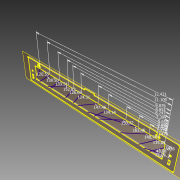
# Autodesk Inventor part: Panel_front
Saved by Autodesk Inventor 2013 (Build 170138000, 138)
## iProperties
Created: 2013-02-02
Part Number: Panel_front
Material: Aluminum 6061
Document SubType Name: Modeling
Designer: xylzlyx
Density: 1 g/cm^3
Author: xylzlyx
Autodesk Inventor part; units mm, degrees
ref_plane "YZ Plane" through (0, 0, 0) normal (1, 0, 0) x (0, 1, 0)
ref_plane "XZ Plane" through (0, 0, 0) normal (0, 1, 0) x (-1, 0, 0)
ref_plane "XY Plane" through (0, 0, 0) normal (0, 0, 1) x (1, 0, 0)
ref_plane "Work Plane1" through (0, 0, -9.525) normal (0, 0, 1) x (1, 0, 0)
sketch "Sketch1" plane through (0, 0, -9.525) normal (0, 0, 1) x (1, 0, 0)
  line L0 (381, -60.8043) -> (381, -64.0283) construction
  line L1 (381, -64.0283) -> (0, -64.0283) construction
  line L2 (0, -64.0283) -> (0, -60.8043) construction
  line L3 (0, -60.8043) -> (381, -60.8043) construction
  line L4 (381, 0) -> (0, 0) construction
  line L5 (0, 0) -> (0, 3.175) construction
  line L6 (0, 3.175) -> (381, 3.175) construction
  line L7 (381, 3.175) -> (381, 0) construction
  line L8 (381, -60.8043) -> (0, -60.8043)
  line L9 (0, -60.8043) -> (0, 0)
  line L10 (0, 0) -> (381, 0)
  line L11 (381, 0) -> (381, -60.8043)
  constraints: 24 end point, 5 horizontal, 4 coincident, 4 vertical, 2 parallel, 1 perpendicular, 8 other
extrude "FrontPanel" add sketch "Sketch1" against normal blind 3.175
fillet "CornerFillet" radius 1 4 edges at (381, -60.8043, -11.1125) (0, -60.8043, -11.1125) (0, 0, -11.1125) (381, 0, -11.1125)
sketch "ScrewSlotSketch" plane through (0, 0, -9.525) normal (0, 0, 1) x (1, 0, 0)
  line L0 (368.3, -28.0035) -> (368.3, -1) projected
  line L1 (12.7, -1) -> (12.7, -28.0035) projected
  line L2 (381, 0) -> (0, 0) construction
  line L3 (0, 0) -> (0, 3.175) construction
  line L4 (0, 3.175) -> (381, 3.175) construction
  line L5 (381, 3.175) -> (381, 0) construction
  line L6 (381, -60.8043) -> (381, -64.0283) construction
  line L7 (381, -64.0283) -> (0, -64.0283) construction
  line L8 (0, -64.0283) -> (0, -60.8043) construction
  line L9 (0, -60.8043) -> (381, -60.8043) construction
  line L10 (344.7987, -8.89) -> (344.7987, 3.175)
  line L11 (344.7987, 3.175) -> (341.0014, 3.175)
  line L12 (341.0014, 3.175) -> (341.0014, -8.89)
  line L13 (341.0014, -8.89) -> (344.7987, -8.89)
  line L14 (346.9958, -8.89) -> (338.8043, -8.89)
  line L15 (338.8043, -8.89) -> (338.8043, -5.8579)
  line L16 (338.8043, -5.8579) -> (346.9958, -5.8579)
  line L17 (346.9958, -5.8579) -> (346.9958, -8.89)
  line L18 (36.2014, -8.89) -> (39.9987, -8.89)
  line L19 (39.9987, -8.89) -> (39.9987, 3.175)
  line L20 (39.9987, 3.175) -> (36.2014, 3.175)
  line L21 (36.2014, 3.175) -> (36.2014, -8.89)
  line L22 (34.0043, -8.89) -> (42.1958, -8.89)
  line L23 (42.1958, -8.89) -> (42.1958, -5.8579)
  line L24 (42.1958, -5.8579) -> (34.0043, -5.8579)
  line L25 (34.0043, -5.8579) -> (34.0043, -8.89)
  point P0 (342.9, 3.175)
  point P1 (342.9, -8.89)
  point P2 (38.1, -8.89)
  point P3 (38.1, 3.175)
  dimension "d4" = 12.065
  dimension "d6" = 3.7973
  dimension "d7" = 25.4
  dimension "d8" = 8.1915
  dimension "d9" = 3.0321
  dimension "d10" = 3.7973
  dimension "d11" = 12.065
  dimension "d12" = 8.1915
  dimension "d13" = 3.0321
  dimension "d14" = 25.4
  constraints: 48 end point, 11 parallel, 6 horizontal, 6 midpoint, 4 vertical, 2 perpendicular, 2 point on line, 1 collinear, 7 other
  measures "d4" distance of L10.start L10.end
  measures "d6" distance of L10.end L11.end
  measures "d7" distance from line of L0 point (342.9, 3.175)
  measures "d8" distance of L14.start L14.end
  measures "d9" distance of L14.end L15.end
  measures "d10" distance of L19.end L20.end
  measures "d11" distance of L20.end L18.start
  measures "d12" distance of L22.start L22.end
  measures "d13" distance of L22.end L23.end
  measures "d14" distance from line of L1 point (38.1, 3.175)
extrude "ScrewSlotExtrusion" cut sketch "ScrewSlotSketch" against normal blind 3.175
fillet "ScrewSlotFillet" radius 0.5 16 edges at (344.7987, 0, -11.1125) (341.0014, 0, -11.1125) (344.7987, -5.8579, -11.1125) (341.0014, -5.8579, -11.1125) (338.8043, -5.8579, -11.1125) (338.8043, -8.89, -11.1125) (346.9958, -8.89, -11.1125) (346.9958, -5.8579, -11.1125) (42.1958, -8.89, -11.1125) (42.1958, -5.8579, -11.1125) (39.9987, -5.8579, -11.1125) (39.9987, 0, -11.1125) (36.2014, 0, -11.1125) (36.2014, -5.8579, -11.1125) (34.0043, -5.8579, -11.1125) (34.0043, -8.89, -11.1125)
sketch "ScrewHoleSketch" plane through (0, 0, -9.525) normal (0, 0, 1) x (1, 0, 0)
  line L0 (34.0043, -8.39) -> (34.0043, -6.3579) projected
  line L1 (368.3, -28.5035) -> (371.475, -28.5035) projected
  line L2 (371.475, -32.3008) -> (368.3, -32.3008) projected
  line L3 (9.525, -28.5035) -> (12.7, -28.5035) projected
  line L4 (12.7, -32.3008) -> (9.525, -32.3008) projected
  line L5 (371.475, -28.5035) -> (371.475, -32.3008) construction
  line L6 (9.525, -28.5035) -> (9.525, -32.3008) construction
  point P0 (0, 0)
  point P1 (11.1125, -30.4021)
  point P2 (369.8875, -30.4021)
  point P3 (369.8875, -28.5035)
  point P4 (371.475, -30.4021)
  point P5 (9.525, -30.4021)
  point P6 (11.1125, -28.5035)
  constraints: 4 end point, 4 midpoint, 2 horizontal alignment, 2 parallel, 2 vertical alignment
hole "ScrewHoles" at (11.1125, -30.4021, -9.525) at (369.8875, -30.4021, -9.525) direction (0, 0, -1) diameter 3.7973 end through all
sketch "BottomTabSketch" plane through (40.4987, 0, -9.525) normal (0, 1, 0) x (1, 0, 0)
  line L0 (162.7014, 3.175) -> (137.3014, 3.175)
  line L1 (137.3014, 3.175) -> (137.3014, 0)
  line L2 (137.3014, 0) -> (162.7014, 0)
  line L3 (162.7014, 0) -> (162.7014, 3.175)
  line L4 (137.0473, 2.929) -> (137.0473, 0.246) projected
  line L5 (137.5473, -0.254) -> (162.4553, -0.254) projected
  point P0 (0, 3.175)
  point P1 (-40.4987, -9.525)
  point P2 (137.3014, 1.5875)
  point P3 (137.0473, 1.5875)
  point P4 (150.0014, 0)
  point P5 (150.0013, -0.254)
  dimension "d29" = 25.4
  constraints: 8 end point, 4 midpoint, 2 horizontal alignment, 2 parallel, 1 horizontal, 1 perpendicular, 1 vertical alignment
  measures "d29" distance of L0.start L0.end
extrude "BottomTab" add sketch "BottomTabSketch" along normal blind 3.175
fillet "BottomTabFillet" radius 0.5 4 edges at (177.8, 0, -11.1125) (177.8, 3.175, -11.1125) (203.2, 3.175, -11.1125) (203.2, 0, -11.1125)
sketch "SlotSketch" plane through (0, 0, -9.525) normal (0, 0, 1) x (1, 0, 0)
  circle A0 centre (11.1125, -30.4021) radius 1.8986 projected
  circle A1 centre (369.8875, -30.4021) radius 1.8986 projected
  line L0 (371.729, -50.6197) -> (368.046, -50.6197)
  line L1 (368.046, -50.6197) -> (368.046, -40.5867)
  line L2 (368.046, -40.5867) -> (371.729, -40.5867)
  line L3 (371.729, -40.5867) -> (371.729, -50.6197)
  line L4 (12.954, -50.6197) -> (9.271, -50.6197)
  line L5 (9.271, -50.6197) -> (9.271, -40.5867)
  line L6 (9.271, -40.5867) -> (12.954, -40.5867)
  line L7 (12.954, -40.5867) -> (12.954, -50.6197)
  line L8 (380, -60.8043) -> (1, -60.8043) projected
  line L9 (203.2, 0.5) -> (203.2, 2.675) projected
  line L10 (11.1125, -30.4021) -> (11.1125, -60.8043) construction
  line L11 (369.8875, -30.4021) -> (369.8875, -60.8043) construction
  point P0 (0, 0)
  point P1 (12.954, -45.6032)
  point P2 (11.1125, -45.6032)
  point P3 (11.1125, -50.6197)
  point P4 (369.8875, -45.6032)
  point P5 (371.729, -45.6032)
  point P6 (369.8875, -50.6197)
  dimension "d34" = 10.033
  dimension "d36" = 3.683
  dimension "d37" = 10.033
  dimension "d38" = 3.683
  constraints: 20 end point, 6 midpoint, 6 parallel, 2 horizontal, 2 horizontal alignment, 2 perpendicular, 2 point on line, 2 vertical alignment
  measures "d34" distance of L0.end L1.end
  measures "d36" distance of L0.start L0.end
  measures "d37" distance of L6.end L4.start
  measures "d38" distance of L4.start L4.end
extrude "Extrusion4" cut sketch "SlotSketch" against normal blind 3.175 contours L0 L1 L2 L3 | L4 L5 L6 L7
fillet "Fillet5" radius 0.5 8 edges at (368.046, -40.5867, -11.1125) (371.729, -40.5867, -11.1125) (371.729, -50.6197, -11.1125) (368.046, -50.6197, -11.1125) (9.271, -40.5867, -11.1125) (12.954, -40.5867, -11.1125) (12.954, -50.6197, -11.1125) (9.271, -50.6197, -11.1125)
sketch "Sketch6" plane through (0, 0, -9.525) normal (0, 0, 1) x (1, 0, 0)
  line L0 (380, -60.8043) -> (1, -60.8043) projected
  line L1 (203.7, 0) -> (340.5014, 0) projected
  circle A0 centre (11.1125, -30.4021) radius 1.8986 projected
  circle A1 centre (369.8875, -30.4021) radius 1.8986 projected
  line L2 (357.1875, -48.1043) -> (23.8125, -48.1043)
  line L3 (23.8125, -48.1043) -> (23.8125, -12.7)
  line L4 (23.8125, -12.7) -> (357.1875, -12.7)
  line L5 (357.1875, -12.7) -> (357.1875, -48.1043)
  point P0 (0, 0)
  dimension "d42" = 12.7
  dimension "d43" = 12.7
  dimension "d44" = 12.7
  dimension "d45" = 12.7
  constraints: 8 end point, 2 parallel, 1 horizontal, 1 perpendicular
  measures "d42" distance from line of L0 L2.start
  measures "d43" distance between parallel lines of L1 L4
  measures "d44" distance from line of A1.centre L5
  measures "d45" distance from line of A0.centre L3
extrude "Extrusion5" cut sketch "Sketch6" against normal blind 25.4 contours L2 L3 L4 L5
fillet "Fillet6" radius 0.5 4 edges at (357.1875, -48.1043, -11.1125) (357.1875, -12.7, -11.1125) (23.8125, -48.1043, -11.1125) (23.8125, -12.7, -11.1125)
sketch "Sketch7" plane through (0, 0, -9.525) normal (0, 0, 1) x (1, 0, 0)
  line L0 (357.1875, -13.2) -> (357.1875, -47.6043) projected
  arc A0 (356.6875, -48.1043) -> (357.1875, -47.6043) centre (356.6875, -47.6043) ccw projected
  line L1 (356.6875, -48.1043) -> (24.3125, -48.1043) projected
  arc A1 (23.8125, -47.6043) -> (24.3125, -48.1043) centre (24.3125, -47.6043) ccw projected
  line L2 (23.8125, -47.6043) -> (23.8125, -13.2) projected
  arc A2 (24.3125, -12.7) -> (23.8125, -13.2) centre (24.3125, -13.2) ccw projected
  line L3 (24.3125, -12.7) -> (356.6875, -12.7) projected
  arc A3 (357.1875, -13.2) -> (356.6875, -12.7) centre (356.6875, -13.2) ccw projected
  line L4 (371.729, -41.0867) -> (371.729, -50.1197) projected
  arc A4 (371.229, -50.6197) -> (371.729, -50.1197) centre (371.229, -50.1197) ccw projected
  line L5 (371.229, -50.6197) -> (368.546, -50.6197) projected
  arc A5 (368.046, -50.1197) -> (368.546, -50.6197) centre (368.546, -50.1197) ccw projected
  line L6 (368.046, -50.1197) -> (368.046, -41.0867) projected
  arc A6 (368.546, -40.5867) -> (368.046, -41.0867) centre (368.546, -41.0867) ccw projected
  line L7 (368.546, -40.5867) -> (371.229, -40.5867) projected
  arc A7 (371.729, -41.0867) -> (371.229, -40.5867) centre (371.229, -41.0867) ccw projected
  line L8 (12.954, -41.0867) -> (12.954, -50.1197) projected
  arc A8 (12.454, -50.6197) -> (12.954, -50.1197) centre (12.454, -50.1197) ccw projected
  line L9 (12.454, -50.6197) -> (9.771, -50.6197) projected
  arc A9 (9.271, -50.1197) -> (9.771, -50.6197) centre (9.771, -50.1197) ccw projected
  line L10 (9.271, -50.1197) -> (9.271, -41.0867) projected
  arc A10 (9.771, -40.5867) -> (9.271, -41.0867) centre (9.771, -41.0867) ccw projected
  line L11 (9.771, -40.5867) -> (12.454, -40.5867) projected
  arc A11 (12.954, -41.0867) -> (12.454, -40.5867) centre (12.454, -41.0867) ccw projected
  arc A12 (203.2, 2.675) -> (202.7, 3.175) centre (202.7, 2.675) ccw projected
  line L12 (178.3, 3.175) -> (202.7, 3.175) projected
  arc A13 (178.3, 3.175) -> (177.8, 2.675) centre (178.3, 2.675) ccw projected
  line L13 (177.8, 0.5) -> (177.8, 2.675) projected
  arc A14 (177.3, 0) -> (177.8, 0.5) centre (177.3, 0.5) ccw projected
  line L14 (40.4987, 0) -> (177.3, 0) projected
  arc A15 (40.4987, 0) -> (39.9987, -0.5) centre (40.4987, -0.5) ccw projected
  line L15 (39.9987, -0.5) -> (39.9987, -5.3579) projected
  arc A16 (39.9987, -5.3579) -> (40.4987, -5.8579) centre (40.4987, -5.3579) ccw projected
  line L16 (40.4987, -5.8579) -> (41.6958, -5.8579) projected
  arc A17 (42.1958, -6.3579) -> (41.6958, -5.8579) centre (41.6958, -6.3579) ccw projected
  line L17 (42.1958, -6.3579) -> (42.1958, -8.39) projected
  arc A18 (41.6958, -8.89) -> (42.1958, -8.39) centre (41.6958, -8.39) ccw projected
  line L18 (41.6958, -8.89) -> (34.5043, -8.89) projected
  arc A19 (34.0043, -8.39) -> (34.5043, -8.89) centre (34.5043, -8.39) ccw projected
  line L19 (34.0043, -8.39) -> (34.0043, -6.3579) projected
  arc A20 (34.5043, -5.8579) -> (34.0043, -6.3579) centre (34.5043, -6.3579) ccw projected
  line L20 (34.5043, -5.8579) -> (35.7014, -5.8579) projected
  arc A21 (35.7014, -5.8579) -> (36.2014, -5.3579) centre (35.7014, -5.3579) ccw projected
  line L21 (36.2014, -5.3579) -> (36.2014, -0.5) projected
  arc A22 (36.2014, -0.5) -> (35.7014, 0) centre (35.7014, -0.5) ccw projected
  line L22 (1, 0) -> (35.7014, 0) projected
  arc A23 (1, 0) -> (0, -1) centre (1, -1) ccw projected
  line L23 (0, -59.8043) -> (0, -1) projected
  arc A24 (0, -59.8043) -> (1, -60.8043) centre (1, -59.8043) ccw projected
  line L24 (380, -60.8043) -> (1, -60.8043) projected
  arc A25 (380, -60.8043) -> (381, -59.8043) centre (380, -59.8043) ccw projected
  line L25 (381, -1) -> (381, -59.8043) projected
  arc A26 (381, -1) -> (380, 0) centre (380, -1) ccw projected
  line L26 (345.2987, 0) -> (380, 0) projected
  arc A27 (345.2987, 0) -> (344.7987, -0.5) centre (345.2987, -0.5) ccw projected
  line L27 (344.7987, -0.5) -> (344.7987, -5.3579) projected
  arc A28 (344.7987, -5.3579) -> (345.2987, -5.8579) centre (345.2987, -5.3579) ccw projected
  line L28 (345.2987, -5.8579) -> (346.4958, -5.8579) projected
  arc A29 (346.9958, -6.3579) -> (346.4958, -5.8579) centre (346.4958, -6.3579) ccw projected
  line L29 (346.9958, -6.3579) -> (346.9958, -8.39) projected
  arc A30 (346.4958, -8.89) -> (346.9958, -8.39) centre (346.4958, -8.39) ccw projected
  line L30 (346.4958, -8.89) -> (339.3043, -8.89) projected
  arc A31 (338.8043, -8.39) -> (339.3043, -8.89) centre (339.3043, -8.39) ccw projected
  line L31 (338.8043, -8.39) -> (338.8043, -6.3579) projected
  arc A32 (339.3043, -5.8579) -> (338.8043, -6.3579) centre (339.3043, -6.3579) ccw projected
  line L32 (339.3043, -5.8579) -> (340.5014, -5.8579) projected
  arc A33 (340.5014, -5.8579) -> (341.0014, -5.3579) centre (340.5014, -5.3579) ccw projected
  line L33 (341.0014, -5.3579) -> (341.0014, -0.5) projected
  arc A34 (341.0014, -0.5) -> (340.5014, 0) centre (340.5014, -0.5) ccw projected
  line L34 (203.7, 0) -> (340.5014, 0) projected
  arc A35 (203.2, 0.5) -> (203.7, 0) centre (203.7, 0.5) ccw projected
  line L35 (203.2, 0.5) -> (203.2, 2.675) projected
  circle A36 centre (11.1125, -30.4021) radius 1.8986 projected
  circle A37 centre (369.8875, -30.4021) radius 1.8986 projected
  line L36 (357.1875, -36.7105) -> (321.9415, -48.1043)
  line L37 (357.1875, -21.5969) -> (332.397, -48.1043)
  line L38 (344.6458, -12.7) -> (309.178, -48.1043)
  line L39 (326.9119, -12.7) -> (268.5984, -48.1043)
  line L40 (304.4629, -12.7) -> (185.3162, -48.1043)
  line L41 (278.4902, -12.7) -> (215.3456, -48.1043)
  line L42 (237.5513, -12.7) -> (203.2, -48.1043)
  line L43 (212.9458, -12.7) -> (157.4642, -48.1043)
  line L44 (168.7522, -12.7) -> (144.5905, -48.1043)
  line L45 (147.217, -12.7) -> (120.8379, -48.1043)
  line L46 (131.8636, -12.7) -> (62.8918, -48.1043)
  line L47 (105.8433, -12.7) -> (72.2367, -48.1043)
  line L48 (74.5284, -12.7) -> (34.5043, -48.1043)
  line L49 (41.1958, -12.7) -> (23.8125, -42.1574)
  point P0 (0, 0)
  dimension "d49" = 23.5105
  dimension "d50" = 8.3969
  dimension "d51" = 72.086
  dimension "d52" = 43.083
  dimension "d53" = 12.0417
  dimension "d54" = 29.7756
  dimension "d55" = 135.051
  dimension "d56" = 148.736
  dimension "d57" = 52.2246
  dimension "d58" = 163.451
  dimension "d59" = 78.1973
  dimension "d60" = 150.721
  dimension "d61" = 119.1362
  dimension "d62" = 134.135
  dimension "d63" = 143.7417
  dimension "d64" = 147.457
  dimension "d65" = 187.9353
  dimension "d66" = 124.312
  dimension "d67" = 209.4705
  dimension "d68" = 126.689
  dimension "d69" = 224.8239
  dimension "d70" = 152.828
  dimension "d71" = 250.8442
  dimension "d72" = 133.508
  dimension "d73" = 282.1591
  dimension "d74" = 138.505
  dimension "d75" = 315.4918
  dimension "d76" = 120.545
  constraints: 28 end point, 3 point on line, 27 other
  measures "d49" vertical distance of A3.centre L36.start
  measures "d50" vertical distance of A3.centre L37.start
  measures "d51" angle of L0 L36
  measures "d52" angle of L0 L37
  measures "d53" distance of A3.end L38.start
  measures "d54" distance of A3.end L39.start
  measures "d55" angle to the sketch x axis of L38
  measures "d56" angle to the sketch x axis of L39
  measures "d57" distance of A3.end L40.start
  measures "d58" angle to the sketch x axis of L40
  measures "d59" distance of A3.end L41.start
  measures "d60" angle to the sketch x axis of L41
  measures "d61" distance of A3.end L42.start
  measures "d62" angle to the sketch x axis of L42
  measures "d63" distance of A3.end L43.start
  measures "d64" angle to the sketch x axis of L43
  measures "d65" distance of A3.end L44.start
  measures "d66" angle to the sketch x axis of L44
  measures "d67" distance of A3.end L45.start
  measures "d68" angle to the sketch x axis of L45
  measures "d69" distance of A3.end L46.start
  measures "d70" angle to the sketch x axis of L46
  measures "d71" distance of A3.end L47.start
  measures "d72" angle to the sketch x axis of L47
  measures "d73" distance of A3.centre L48.start
  measures "d74" angle to the sketch x axis of L48
  measures "d75" distance of A3.centre L49.start
  measures "d76" angle to the sketch x axis of L49
equation "\"d4\" = ScrewLen"
equation "\"d6\" = ScrewHoleD"
equation "\"d7\" = ScrewHoleDist"
equation "\"d8\" = NutFlatsGap"
equation "\"d9\" = NutHeightGap"
equation "\"d10\" = ScrewHoleD"
equation "\"d11\" = ScrewLen"
equation "\"d12\" = NutFlatsGap"
equation "\"d13\" = NutHeightGap"
equation "\"d14\" = ScrewHoleDist"
equation "\"d21\" = SlotFilletRad"
equation "\"d22\" = ScrewHoleD"
equation "\"d29\" = TabLength"
equation "\"d33\" = SlotFilletRad"
equation "\"d34\" = SmallSlotLength"
equation "\"d36\" = SlotWidth"
equation "\"d37\" = SmallSlotLength"
equation "\"d38\" = SlotWidth"
equation "\"d41\" = SlotFilletRad"
equation "\"d42\" = EdgeThickness"
equation "\"d43\" = EdgeThickness"
equation "\"d44\" = EdgeThickness"
equation "\"d45\" = EdgeThickness"
equation "\"d48\" = SlotFilletRad"
equation "\"ScrewLen\" = 12.065"
equation "\"ScrewHoleD\" = 3.7973"
equation "\"NutFlatsGap\" = 8.1915"
equation "\"NutHeightGap\" = 3.032125"
equation "\"SlotFilletRad\" = 0.5"
equation "\"TabLength\" = 25.4"
equation "\"SmallSlotLength\" = 10.033"
equation "\"SlotWidth\" = 3.683"
equation "\"EdgeThickness\" = 12.7"
equation "\"ScrewHoleDist\" = 25.4"
body "Solid1"
